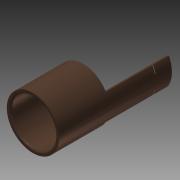
# Autodesk Inventor part: ConnectorSocket
Saved by Autodesk Inventor 2014 SP2 (Build 180246200, 246)
## iProperties
Created: 2015-09-20
Part Number: ConnectorSocket
Material: Generic
Document SubType Name: Modeling
Designer: Lukasz Szmit
Density: 1 g/cm^3
Appearance: Default
Mass: 0.615332 g
Surface Area: 13.4344 cm^2
Volume: 0.615332 cm^3
Author: Lukasz Szmit
Autodesk Inventor part; units mm, degrees
sketch "Sketch1" plane through (0, 0, 0) normal (0, 0, 1) x (1, 0, 0)
  line L0 (-6.25, -13.5) -> (-6.75, -13.5)
  line L1 (-6.75, -13.5) -> (-6.75, 15.5)
  line L2 (-6.25, 16) -> (-6.25, 16)
  line L3 (-5.75, 15.5) -> (-5.75, -13)
  arc A0 (-6.25, -13.5) -> (-5.75, -13) centre (-6.25, -13) ccw
  arc A1 (-6.25, 16) -> (-6.75, 15.5) centre (-6.25, 15.5) ccw
  arc A2 (-5.75, 15.5) -> (-6.25, 16) centre (-6.25, 15.5) ccw
  line L4 (0, -19.545) -> (0, 22.045) projected
  point P0 (-5.75, -13.5)
  point P1 (-6.75, 16)
  point P2 (0, 0)
  dimension "d2" = 29.5
  dimension "d3" = 1
  dimension "d4" = 5.75
  dimension "d5" = 13.5
  dimension "d6" = 0.5
  constraints: 8 end point, 6 point on circle, 6 tangent, 4 point on line, 3 centre point, 2 equal radius, 2 perpendicular, 1 parallel, 1 other
  measures "d2" distance of L0.end point (-6.75, 16)
  measures "d3" distance of point (-5.75, -13.5) L0.end
  measures "d4" distance from line of point (0, 0) L3
  measures "d5" distance from line of point (0, 0) L0
  measures "d6" radius of A0
revolve "Revolution1" add sketch "Sketch1" angle 360 about axis through (0, -10, 0) along (0, 1, 0)
ref_plane "Work Plane1" through (0, 15.5, 0) normal (0, 1, 0) x (-1, 0, 0)
sketch "Sketch3" plane through (0, 15.5, 0) normal (0, 1, 0) x (-1, 0, 0)
  circle A0 centre (0, 0) radius 6.75 construction
  circle A1 centre (0, 0) radius 5.75 construction
  arc A2 (-5.8328, -3.3972) -> (-5.8584, 3.3528) centre (0, 0) ccw
  arc A3 (-4.9687, -2.8939) -> (-4.9905, 2.8561) centre (0, 0) ccw
  line L0 (-0.0608, 0.0348) -> (-0.0605, -0.0352)
  line L1 (0, 0) -> (-0.0608, 0.0348)
  line L2 (-4.9905, 2.8561) -> (-5.8584, 3.3528)
  line L3 (0, 0) -> (-0.0605, -0.0352)
  line L4 (-4.9687, -2.8939) -> (-5.8328, -3.3972)
  point P0 (-0.0584, 6.7497)
  point P1 (-0.0071, -6.75)
  point P2 (-0.0546, 5.7497)
  point P3 (-0.0085, -5.75)
  dimension "d22" = 60
  constraints: 10 end point, 10 point on circle, 2 centre point, 2 coincident
  measures "d22" angle of L4 L2
ref_plane "Work Plane3" through (5.8328, -0.5, -3.3972) normal (-0.5032861, 0, -0.8641199) x (-0.8641199, 0, 0.5032861)
sketch "Sketch4" plane through (5.8328, -0.5, -3.3972) normal (-0.5032861, 0, -0.8641199) x (-0.8641199, 0, 0.5032861)
  arc A0 (1, 16) -> (0, 16) centre (0.5, 16) ccw construction
  line L0 (0, 0) -> (0, 16) construction
  line L1 (1, 16) -> (1, 0) construction
  line L2 (0, 12.15) -> (1, 12.15)
  line L3 (1, 12.15) -> (1, 12)
  line L4 (1, 12) -> (0, 12)
  line L5 (0, 12) -> (0, 12.15)
  line L6 (6.75, -18.9) -> (6.75, 22.4) projected
  point P0 (6.75, 0.5)
  dimension "d14" = 1
  dimension "d15" = 0.15
  dimension "d16" = 4.5
  constraints: 8 end point, 2 point on line
  measures "d14" distance of L3.end L4.end
  measures "d15" distance of L4.end L2.start
revolve "Revolution2" cut sketch "Sketch4" angle 15 about axis through (0, -10, 0) along (0, -1, 0)
ref_plane "Work Plane2" through (4.9905, -0.5, 2.8561) normal (-0.4967067, 0, 0.8679184) x (0.8679184, 0, 0.4967067)
sketch "Sketch5" plane through (4.9905, -0.5, 2.8561) normal (-0.4967067, 0, 0.8679184) x (0.8679184, 0, 0.4967067)
  arc A0 (1, 16) -> (0, 16) centre (0.5, 16) ccw construction
  line L0 (0, 0) -> (0, 16) construction
  line L1 (1, 16) -> (1, 0) construction
  line L2 (0, 12.15) -> (1, 12.15)
  line L3 (1, 12.15) -> (1, 12)
  line L4 (1, 12) -> (0, 12)
  line L5 (0, 12) -> (0, 12.15)
  line L6 (6.75, -18.9) -> (6.75, 22.4)
  line L7 (-5.75, -27.16) -> (-5.75, 30.66) projected
  point P0 (-5.75, 0.5)
  point P1 (6.75, 0.5)
  dimension "d18" = 1
  dimension "d19" = 0.15
  dimension "d20" = 4.5
  constraints: 14 end point, 2 point on circle, 2 point on line, 1 centre point
  measures "d18" distance of L3.end L4.end
  measures "d19" distance of L4.end L2.start
revolve "Revolution3" cut sketch "Sketch5" angle 15 about axis through (0, -10, 0) along (0, 1, 0)
extrude "Extrusion2" cut sketch "Sketch3" along normal blind 0.5 and the other way blind 16 contours L4 A3 L2 A2
body "Solid1"
